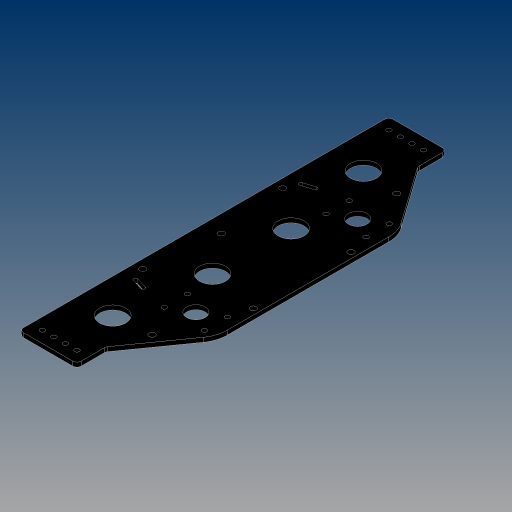
# Autodesk Inventor part: ELEV_027_GEARBOX1
Saved by Autodesk Inventor 2024.3 (Build 283343000, 343)
## iProperties
Created: 2024-12-02
Part Number: ELEV_027_GEARBOX1
Material: Aluminum 6061
Document SubType Name: Modeling
Designer: Kenji
Density: 2.7 g/cm^3
Appearance: Anodized - Black
Mass: 464.349 g
Surface Area: 813.217 cm^2
Volume: 171.981 cm^3
Author: Kenji
Autodesk Inventor part; units mm, degrees
ref_plane "YZ Plane" through (0, 0, 0) normal (1, 0, 0) x (0, 1, 0)
ref_plane "XZ Plane" through (0, 0, 0) normal (0, 1, 0) x (-1, 0, 0)
ref_plane "XY Plane" through (0, 0, 0) normal (0, 0, 1) x (1, 0, 0)
sketch "Sketch1" plane through (0, 0, 0) normal (0, 1, 0) x (-1, 0, 0)
  line L0 (0, 0) -> (63.5, 0) construction
  line L1 (63.5, 0) -> (63.5, -25.4) construction
  line L2 (63.5, -25.4) -> (0, -25.4) construction
  line L3 (0, -25.4) -> (0, 0) construction
  line L4 (0, -381) -> (63.5, -381) construction
  line L5 (63.5, -381) -> (63.5, -406.4) construction
  line L6 (63.5, -406.4) -> (0, -406.4) construction
  line L7 (0, -406.4) -> (0, -381) construction
  circle A0 centre (26.0346, -341.0966) radius 22.733 construction
  circle A1 centre (26.0346, -65.3034) radius 22.733 construction
  line L8 (26.0346, -65.3034) -> (26.0346, -341.0966) construction
  line L9 (63.5, -203.2) -> (-50.8, -203.2) construction
  circle A2 centre (26.0346, -65.3034) radius 14.2875
  circle A3 centre (26.0346, -341.0966) radius 14.2875
  circle A4 centre (26.0346, -65.3034) radius 27.2288 construction
  circle A5 centre (26.0346, -341.0966) radius 27.2288 construction
  circle A6 centre (692.1496, -341.0966) radius 22.733 construction
  circle A7 centre (692.1496, -341.0966) radius 27.2288 construction
  line L10 (-50.8, 0) -> (-50.8, -406.4) construction
  circle A8 centre (-16.5354, -292.1) radius 31.7246 construction
  circle A9 centre (-16.5354, -114.3) radius 31.7246 construction
  circle A10 centre (-16.5354, -292.1) radius 10.16 construction
  circle A11 centre (-16.5354, -114.3) radius 10.16 construction
  circle A12 centre (-16.5354, -292.1) radius 10.16
  circle A13 centre (-16.5354, -114.3) radius 10.16
  line L11 (692.1496, -363.8296) -> (26.0346, -363.8296) construction
  line L12 (-48.26, -114.3) -> (-50.8, -114.3) construction
  line L13 (63.5, -25.4) -> (63.5, -381) construction
  line L14 (-48.26, -292.1) -> (-50.8, -292.1) construction
  circle A14 centre (10.9389, -160.02) radius 43.18 construction
  circle A15 centre (10.9389, -160.02) radius 45.72 construction
  circle A16 centre (10.9389, -246.38) radius 43.18 construction
  line L15 (10.9389, -160.02) -> (10.9389, -246.38) construction
  circle A17 centre (10.9389, -160.02) radius 14.2875
  circle A18 centre (10.9389, -246.38) radius 14.2875
  circle A19 centre (10.9389, -246.38) radius 45.72 construction
  line L16 (10.9389, -203.2) -> (63.5, -203.2) construction
  circle A20 centre (10.9389, -160.02) radius 14.3256 construction
  circle A21 centre (26.0346, -65.3034) radius 28.6512 construction
  circle A22 centre (26.0346, -341.0966) radius 28.6512 construction
  circle A23 centre (10.9389, -246.38) radius 14.3256 construction
  line L17 (53.3378, -73.9883) -> (24.5905, -164.3625) construction
  line L18 (-2.6157, -65.0706) -> (-3.3862, -159.9036) construction
  line L19 (53.3378, -332.4117) -> (24.5905, -242.0375) construction
  line L20 (-3.3862, -246.4964) -> (-2.6157, -341.3294) construction
  circle A24 centre (12.7, -12.7) radius 2.54
  line L21 (63.5, -12.7) -> (0, -12.7) construction
  circle A25 centre (25.4, -12.7) radius 2.54
  circle A26 centre (38.1, -12.7) radius 2.54
  circle A27 centre (50.8, -12.7) radius 2.54
  circle A28 centre (12.7, -393.7) radius 2.54
  circle A29 centre (25.4, -393.7) radius 2.54
  circle A30 centre (38.1, -393.7) radius 2.54
  circle A31 centre (50.8, -393.7) radius 2.54
  line L22 (63.5, -401.6375) -> (63.5, -4.7625)
  line L23 (58.7375, 0) -> (4.7625, 0)
  line L24 (0, -4.7625) -> (0, -25.4)
  circle A32 centre (-16.5354, -114.3) radius 34.2646 construction
  line L25 (0, 0) -> (-50.8, 0) construction
  line L26 (-50.8, 0) -> (-50.8, -25.4) construction
  line L27 (-50.8, -25.4) -> (0, -25.4) construction
  line L28 (0, -25.4) -> (0, 0) construction
  line L29 (0, -25.4) -> (0, -30.2327)
  line L30 (-0.8777, -32.9877) -> (-44.4852, -94.479)
  arc A33 (-0.8777, -32.9877) -> (0, -30.2327) centre (-4.7625, -30.2327) ccw
  circle A34 centre (-16.5354, -292.1) radius 34.2646 construction
  line L31 (-50.8, -114.3) -> (-50.8, -292.1)
  line L32 (58.7375, -406.4) -> (4.7625, -406.4)
  line L33 (0, -381) -> (0, -401.6375)
  line L34 (0, -381) -> (0, -376.1673)
  line L35 (-0.8777, -373.4123) -> (-44.4852, -311.921)
  arc A35 (0, -376.1673) -> (-0.8777, -373.4123) centre (-4.7625, -376.1673) ccw
  arc A36 (-44.4852, -94.479) -> (-50.8, -114.3) centre (-16.5354, -114.3) ccw
  arc A37 (-50.8, -292.1) -> (-44.4852, -311.921) centre (-16.5354, -292.1) ccw
  arc A38 (4.7625, 0) -> (0, -4.7625) centre (4.7625, -4.7625) ccw
  arc A39 (63.5, -4.7625) -> (58.7375, 0) centre (58.7375, -4.7625) ccw
  arc A40 (58.7375, -406.4) -> (63.5, -401.6375) centre (58.7375, -401.6375) ccw
  arc A41 (0, -401.6375) -> (4.7625, -406.4) centre (4.7625, -401.6375) ccw
  circle A42 centre (47.8399, -112.2206) radius 6.35 construction
  circle A43 centre (47.8399, -112.2206) radius 3.175 construction
  line L36 (47.8399, -112.2206) -> (41.7887, -110.2957) construction
  circle A44 centre (47.8399, -112.2206) radius 1.9844 construction
  line L37 (47.8399, -112.2206) -> (35.7374, -108.3709) construction
  circle A45 centre (35.7374, -108.3709) radius 1.9844 construction
  line L38 (48.4414, -110.3296) -> (36.3389, -106.4799)
  line L39 (47.2384, -114.1116) -> (35.1359, -110.2619)
  arc A46 (47.2384, -114.1116) -> (48.4414, -110.3296) centre (47.8399, -112.2206) ccw
  arc A47 (36.3389, -106.4799) -> (35.1359, -110.2619) centre (35.7374, -108.3709) ccw
  line L40 (48.4414, -296.0704) -> (36.3389, -299.9201)
  line L41 (47.2384, -292.2884) -> (35.1359, -296.1381)
  arc A48 (48.4414, -296.0704) -> (47.2384, -292.2884) centre (47.8399, -294.1794) ccw
  arc A49 (35.1359, -296.1381) -> (36.3389, -299.9201) centre (35.7374, -298.0291) ccw
  circle A50 centre (44.3715, -203.2) radius 6.35 construction
  circle A51 centre (53.8397, -126.2299) radius 6.35 construction
  circle A52 centre (-13.904, -68.6812) radius 6.35 construction
  circle A53 centre (-44.45, -149.4985) radius 6.35 construction
  line L42 (-33.9779, -151.4878) -> (-38.2116, -150.6836) construction
  line L43 (-37.8265, -141.1468) -> (-40.5043, -144.5232) construction
  circle A54 centre (-44.45, -149.4985) radius 3.2512
  line L44 (-2.5147, -67.718) -> (-7.5766, -68.1461) construction
  line L45 (-14.2697, -75.0207) -> (-14.5622, -80.0923) construction
  circle A55 centre (-13.904, -68.6812) radius 3.2512
  line L46 (51.3398, -120.3927) -> (50.3398, -118.0578) construction
  line L47 (48.8512, -130.1589) -> (46.8559, -131.7306) construction
  line L48 (40.484, -198.1791) -> (38.929, -196.1707) construction
  line L49 (40.484, -208.2209) -> (38.929, -210.2293) construction
  circle A56 centre (53.8397, -126.2299) radius 3.2512
  circle A57 centre (44.3715, -203.2) radius 3.2512
  circle A58 centre (53.8397, -280.1701) radius 6.35 construction
  circle A59 centre (-13.904, -337.7188) radius 6.35 construction
  circle A60 centre (-44.45, -256.9015) radius 6.35 construction
  circle A61 centre (-44.45, -256.9015) radius 3.2512
  circle A62 centre (-13.904, -337.7188) radius 3.2512
  circle A63 centre (53.8397, -280.1701) radius 3.2512
  circle A64 centre (-16.5354, -114.3) radius 25.4 construction
  circle A65 centre (-16.5354, -88.9) radius 2.54 construction
  circle A66 centre (-29.2354, -92.303) radius 2.54 construction
  circle A67 centre (-38.5324, -101.6) radius 2.54
  circle A68 centre (-41.9354, -114.3) radius 2.54 construction
  circle A69 centre (-38.5324, -127) radius 2.54
  circle A70 centre (-29.2354, -136.297) radius 2.54 construction
  circle A71 centre (-16.5354, -139.7) radius 2.54 construction
  circle A72 centre (-3.8354, -136.297) radius 2.54 construction
  circle A73 centre (5.4616, -127) radius 2.54
  circle A74 centre (8.8646, -114.3) radius 2.54 construction
  circle A75 centre (5.4616, -101.6) radius 2.54
  circle A76 centre (-3.8354, -92.303) radius 2.54 construction
  circle A77 centre (-16.5354, -317.5) radius 2.54 construction
  circle A78 centre (-38.5324, -304.8) radius 2.54
  circle A79 centre (-38.5324, -279.4) radius 2.54
  circle A80 centre (-16.5354, -266.7) radius 2.54 construction
  circle A81 centre (5.4616, -279.4) radius 2.54
  circle A82 centre (5.4616, -304.8) radius 2.54
  point P0 (0, -31.75)
  point P1 (0, -374.65)
  dimension "d18" = 63.4492
  dimension "d26" = 63.4492
  dimension "d77" = 12.7
  dimension "d93" = 50.8
  dimension "d0" = 25.4
  dimension "d1" = 63.5
  dimension "d2" = 406.4
  dimension "d3" = 45.466
  dimension "d4" = 65.3034
  dimension "d5" = 203.2
  dimension "d6" = 28.575
  dimension "d7" = 54.4576
  dimension "d13" = 692.1496
  dimension "d14" = 50.8
  dimension "d19" = 20.32
  dimension "d33" = 20.32
  dimension "d34" = 666.115
  dimension "d35" = 2.54
  dimension "d48" = 2.54
  dimension "d49" = 86.36
  dimension "d50" = 28.575
  dimension "d51" = 28.575
  dimension "d52" = 43.18
  dimension "d53" = 177.8
  dimension "d54" = 177.8
  dimension "d56" = 57.3024
  dimension "d58" = 28.6512
  dimension "d59" = 12.7
  dimension "d60" = 5.08
  dimension "d63" = 12.7
  dimension "d68" = 2.54
  dimension "d69" = 25.4
  dimension "d70" = 6.35
  dimension "d71" = 4.7625
  dimension "d72" = 2.54
  dimension "d73" = 6.35
  dimension "d74" = 4.7625
  dimension "d75" = 4.7625
  dimension "d76" = 4.7625
  dimension "d78" = 6.35
  dimension "d81" = 38.1
  dimension "d83" = 3.9688
  dimension "d84" = 12.7
  dimension "d85" = 12.7
  dimension "d86" = 6.5024
  dimension "d87" = 5.08
  dimension "d88" = 6.5024
  dimension "d89" = 2.54
  dimension "d90" = 6.5024
  dimension "d91" = 2.54
  dimension "d92" = 6.5024
  dimension "d94" = 5.08
  dimension "d97" = 360
  constraints: 100 end point, 76 centre point, 53 point on circle, 40 point on line, 31 tangent, 26 coincident, 22 symmetric about line, 15 equal radius, 7 horizontal, 7 parallel, 7 perpendicular, 6 collinear, 6 equal length, 6 midpoint, 6 vertical, 4 vertical alignment, 3 concentric, 3 horizontal alignment, 69 other
  measures "d0" distance between parallel lines of L0 L2
  measures "d1" distance of L0.start L0.end
  measures "d2" distance between parallel lines of L6 L0
  measures "d3" diameter of A1
  measures "d4" distance from line of L6 L8.end
  measures "d5" distance between parallel lines of L6 L9
  measures "d6" diameter of A2
  measures "d7" diameter of A4
  measures "d13" distance from line of L7 point (692.15, -341.097)
  measures "d14" distance between parallel lines of L10 L7
  measures "d19" diameter of A10
  measures "d33" diameter of A13
  measures "d34" distance of L11.start L11.end
  measures "d35" distance of L12.start L12.end
  measures "d48" radial gap between concentric circles of A14 A15
  measures "d49" diameter of A14
  measures "d50" diameter of A17
  measures "d51" diameter of A18
  measures "d52" distance from line of L15.start L16
  measures "d53" distance between parallel lines of L4 L16
  measures "d54" distance of A34.centre A32.centre
  measures "d56" diameter of A21
  measures "d58" diameter of A20
  measures "d59" distance from line of L3 A24.centre
  measures "d60" diameter of A24
  measures "d63" distance of A24.centre A25.centre
  measures "d69" distance between parallel lines of L25 L27
  measures "d70" distance of L27.end point (0, -31.75)
  measures "d71" radius of A33
  measures "d73" distance of L4.start point (0, -374.65)
  measures "d74" radius of A35
  measures "d75" radius of A38
  measures "d76" radius of A39
  measures "d78" diameter of A43
  measures "d81" distance of L36.end L17.start
  measures "d83" diameter of A44
  measures "d84" distance of L37.start L37.end
  measures "d85" diameter of A50
  measures "d86" diameter of A54
  measures "d87" distance of L44.start L44.end
  measures "d88" diameter of A55
  measures "d89" distance of L46.start L46.end
  measures "d90" diameter of A56
  measures "d91" distance of L48.start L48.end
  measures "d92" diameter of A57
  measures "d94" diameter of A65
extrude "Extrusion1" add sketch "Sketch1" along normal blind 4.7625
body "Solid1"
